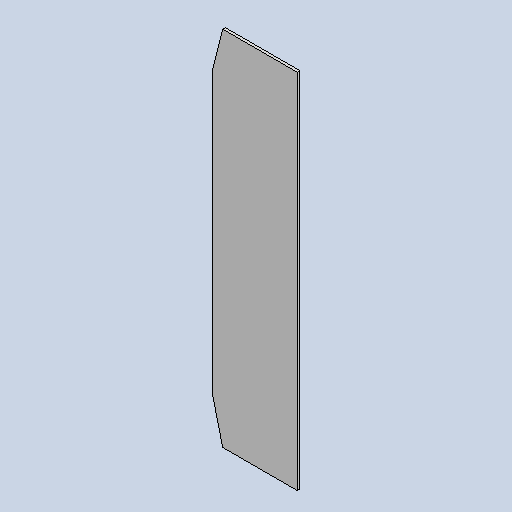
# Autodesk Inventor part: Angle changer polycarb
Saved by Autodesk Inventor 2023.2 (Build 272271030, 271C)
## iProperties
Created: 2023-04-03
Part Number: Angle changer polycarb
Material: Generic
Document SubType Name: Modeling
Designer: Main Account
Density: 1 g/cm^3
Appearance: Default
Author: Main Account
Autodesk Inventor part; units mm, degrees
ref_plane "YZ Plane" through (0, 0, 0) normal (1, 0, 0) x (0, 1, 0)
ref_plane "XZ Plane" through (0, 0, 0) normal (0, 1, 0) x (-1, 0, 0)
ref_plane "XY Plane" through (0, 0, 0) normal (0, 0, 1) x (1, 0, 0)
sketch "Sketch1" plane through (0, 0, 0) normal (0, 0, 1) x (1, 0, 0)
  line L0 (3.9874, -107.95) -> (-5.3154, -107.95) construction
  line L1 (6.3686, -83.7157) -> (6.3686, -107.95) construction
  line L2 (6.3686, -107.95) -> (-38.0814, -107.95)
  line L3 (-44.4314, -82.55) -> (-44.4314, 82.55)
  line L4 (-38.0814, 107.95) -> (6.3686, 107.95)
  line L5 (6.3686, 107.95) -> (6.3686, -107.95)
  line L6 (-44.4314, -107.95) -> (-38.0814, -107.95) construction
  line L7 (-44.4314, -107.95) -> (-44.4314, -82.55) construction
  line L8 (-44.4314, 107.95) -> (-38.0814, 107.95) construction
  line L9 (-44.4314, 107.95) -> (-44.4314, 82.55) construction
  line L10 (-38.0814, 107.95) -> (-44.4314, 82.55)
  line L11 (-44.4314, -82.55) -> (-38.0814, -107.95)
  point P0 (0, 0)
  dimension "d0" = 50.8
  dimension "d1" = 215.9
  dimension "d2" = 6.35
  dimension "d3" = 25.4
  dimension "d4" = 6.35
  dimension "d5" = 25.4
  constraints: 24 end point, 2 horizontal, 2 parallel, 1 perpendicular, 1 vertical
  measures "d0" distance of L8.start L4.end
  measures "d1" distance of L6.start L8.start
  measures "d2" distance of L2.end L6.start
  measures "d3" distance of L3.start L6.start
  measures "d4" distance of L4.start L8.start
  measures "d5" distance of L3.end L8.start
extrude "Extrusion1" add sketch "Sketch1" along normal blind 1.5875
body "Solid1"
